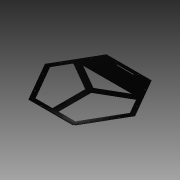
# Autodesk Inventor part: top
Saved by Autodesk Inventor 2015 SP1 (Build 190203100, 203)
## iProperties
Created: 2015-04-18
Part Number: top
Material: Ogólny
Document SubType Name: Konstrukcja blachowa
Designer: Marcin
Density: 1 g/cm^3
Sheet Metal Rule: Domyślny
Appearance: Gładki - czarny
Author: Marcin
Autodesk Inventor part; units mm, degrees
ref_plane "YZ Plane" through (0, 0, 0) normal (1, 0, 0) x (0, 1, 0)
ref_plane "XZ Plane" through (0, 0, 0) normal (0, 1, 0) x (-1, 0, 0)
ref_plane "XY Plane" through (0, 0, 0) normal (0, 0, 1) x (1, 0, 0)
sketch "Szkic1" plane through (0, 0, 0) normal (0, 0, 1) x (1, 0, 0)
  line L0 (76.2102, 132) -> (152.4205, 0)
  line L1 (152.4205, 0) -> (76.2102, -132)
  line L2 (76.2102, -132) -> (-76.2102, -132)
  line L3 (-76.2102, -132) -> (-152.4205, 0)
  line L4 (-152.4205, 0) -> (-76.2102, 132)
  line L5 (-76.2102, 132) -> (76.2102, 132)
  point P0 (0, 0)
  point P1 (0, 0)
  dimension "d0" = 132
  measures "d0" distance from line of L5 point (0, 0)
extrude "Płyta1" add sketch "Szkic1" along normal blind 0.8
sketch "Szkic2" plane through (0, 0, 0.8) normal (0, 0, 1) x (1, 0, 0)
  line L0 (152.4205, 0) -> (76.2102, -132) projected
  line L1 (76.2102, 132) -> (152.4205, 0) projected
  line L2 (-76.2102, 132) -> (76.2102, 132) projected
  line L3 (-152.4205, 0) -> (-76.2102, 132) projected
  line L4 (-76.2102, -132) -> (-152.4205, 0) projected
  line L5 (76.2102, -132) -> (-76.2102, -132) projected
  line L6 (0, 132) -> (0, -132) construction
  line L7 (-21.7321, -117) -> (-67.55, -117)
  line L8 (-67.55, -117) -> (-135.1, 0)
  line L9 (-36.5957, 60) -> (-100.4589, 60)
  line L10 (-100.4589, 60) -> (-135.1, 0)
  line L11 (-152.4205, 0) -> (-76.2102, 132) projected
  line L12 (21.7321, -117) -> (67.55, -117)
  line L13 (67.55, -117) -> (135.1, 0)
  line L14 (36.5957, 60) -> (100.4589, 60)
  line L15 (100.4589, 60) -> (135.1, 0)
  line L16 (-36.5957, 60) -> (0, 60)
  line L17 (0, 60) -> (36.5957, 60)
  line L18 (-21.7321, -117) -> (21.7321, -117)
  point P0 (0, 0)
  dimension "d5" = 15
  dimension "d6" = 15
  dimension "d7" = 15
  dimension "d14" = 177
  constraints: 24 end point, 5 symmetric about line, 4 parallel, 2 horizontal, 2 midpoint, 1 collinear, 1 point on line
  measures "d5" distance between parallel lines of L3 L10
  measures "d6" distance between parallel lines of L8 L4
  measures "d7" distance between parallel lines of L7 L5
  measures "d14" distance between parallel lines of L14 L12
extrude "Wytnij3" cut sketch "Szkic2" against normal blind 0.8 contours L7 L8 L10 L9 L16 L17 L14 L15 L13 L12 L18
sketch "Szkic3" plane through (0, 0, 0.8) normal (0, 0, 1) x (1, 0, 0)
  line L0 (135.1, 0) -> (67.55, -117)
  line L1 (-67.55, -117) -> (-135.1, 0)
  line L2 (67.55, -117) -> (-67.55, -117)
  line L3 (100.4589, 60) -> (135.1, 0)
  line L4 (-135.1, 0) -> (-100.4589, 60)
  line L5 (67.55, -117) -> (135.1, 0) construction
  line L6 (0, 0) -> (0, -117) construction
  line L7 (0, 0) -> (101.325, 58.5) construction
  line L8 (135.1, 0) -> (100.4589, 60) construction
  line L9 (0, 0) -> (-101.325, 58.5) construction
  line L10 (0, 0) -> (-101.325, 58.5) construction
  line L11 (5, 8.6603) -> (-96.325, 67.1603)
  line L12 (-106.325, 49.8397) -> (-5, -8.6603)
  arc A0 (-5, -8.6603) -> (5, 8.6603) centre (0, 0) ccw
  arc A1 (-96.325, 67.1603) -> (-106.325, 49.8397) centre (-101.325, 58.5) ccw
  line L13 (0, 0) -> (0, -117) construction
  line L14 (0, 0) -> (0, -117) construction
  line L15 (-10, 0) -> (-10, -117)
  line L16 (10, -117) -> (10, 0)
  arc A2 (10, 0) -> (-10, 0) centre (0, 0) ccw
  arc A3 (-10, -117) -> (10, -117) centre (0, -117) ccw
  line L17 (0, 0) -> (101.325, 58.5) construction
  line L18 (0, 0) -> (101.325, 58.5) construction
  line L19 (5, -8.6603) -> (106.325, 49.8397)
  line L20 (96.325, 67.1603) -> (-5, 8.6603)
  arc A4 (-5, 8.6603) -> (5, -8.6603) centre (0, 0) ccw
  arc A5 (106.325, 49.8397) -> (96.325, 67.1603) centre (101.325, 58.5) ccw
  point P0 (-50.6625, 29.25)
  point P1 (0, -58.5)
  point P2 (50.6625, 29.25)
  dimension "d15" = 20
  dimension "d18" = 240
  measures "d15" diameter of A1
sheet face with bend "Powierzchnia2" sketch "Szkic3" thickness 0.8 toward (0, 0, -1) bend radius 0.8 relief tear relief width 0.8 relief depth 0.4 contours L19 L16 A0 L11 L20 A5 | A3 L2 | L2 L15 L12 A0 L19 L16 | L19 A0 L16 | A0 A4 A2 | L20 A2 L15 L12 A1 L11 | L11 A2 L20 | L15 A4 L12
bend "Gięcie1"
sketch "Szkic5" plane through (0, 0, 0.8) normal (0, 0, 1) x (1, 0, 0)
  circle A0 centre (-128.0424, -30.624) radius 2 projected
  circle A1 centre (-90.5424, -95.576) radius 2 projected
  point P0 (0, 0)
  point P1 (-37.5, -126.2)
  point P2 (37.5, -126.2)
  point P3 (90.5424, -95.576)
  point P4 (128.0424, -30.624)
  point P5 (128.0424, 30.624)
  point P6 (90.5424, 95.576)
  point P7 (37.5, 126.2)
  point P8 (-37.5, 126.2)
  point P9 (-90.5424, 95.576)
  point P10 (-128.0424, 30.624)
  dimension "d38" = 360
  constraints: 2 coincident, 13 other
hole "Otwór3" at (-128.0424, -30.624, 0.8) at (-90.5424, -95.576, 0.8) at (-37.5, -126.2, 0.8) at (37.5, -126.2, 0.8) at (90.5424, -95.576, 0.8) at (128.0424, -30.624, 0.8) at (128.0424, 30.624, 0.8) at (90.5424, 95.576, 0.8) at (37.5, 126.2, 0.8) at (-37.5, 126.2, 0.8) at (-90.5424, 95.576, 0.8) at (-128.0424, 30.624, 0.8) direction (0, 0, -1) diameter 3 depth 0.8 tip angle 118
sketch "Szkic6" plane through (0, 0, 0.8) normal (0, 0, 1) x (1, 0, 0)
  line L0 (28.5, 120.2073) -> (-28.5, 120.2073) projected
  line L1 (-28.5, 120.2073) -> (-28.5, 118.2073) projected
  line L2 (28.5, 118.2073) -> (-28.5, 118.2073) projected
  line L3 (28.5, 120.2073) -> (28.5, 118.2073) projected
  line L4 (-29, 117.7073) -> (-29, 120.7073)
  line L5 (-29, 120.7073) -> (29, 120.7073)
  line L6 (29, 120.7073) -> (29, 117.7073)
  line L7 (29, 117.7073) -> (-29, 117.7073)
  point P0 (0, 0)
  dimension "d54" = 0.5
  constraints: 8 end point, 3 other
  measures "d54" distance between parallel lines of L1 L4
extrude "Wytnij4" cut sketch "Szkic6" against normal blind 0.8 contours L3 L2 L1 L0 | L4 L5 L6 L7
equation "\"d12\" = Grubość"
equation "\"d52\" = Grubość"
equation "\"d55\" = Grubość"
equation "\"d20\" = PromieńGięcia"
equation "\"d21\" = SzerokośćGięciaPodcięcia"
equation "\"d23\" = MinimalnaPozostałość"
equation "\"d22\" = GłębokośćGięciaPodcięcia"
equation "\"d24\" = PromieńGięcia"
equation "\"PromieńGięcia\" = Grubość"
equation "\"SzerokośćGięciaPodcięcia\" = Grubość"
equation "\"GłębokośćGięciaPodcięcia\" = 0.5 * Grubość"
equation "\"RozmiarPodcięciaNarożnika\" = 4 * Grubość"
equation "\"MinimalnaPozostałość\" = 2 * Grubość"
equation "\"PromieńPrzejścia\" = PromieńGięcia"
equation "\"Rozmiar_promienia_Jacobiego\" = Grubość"
equation "\"Wielk_odstępu\" = Grubość"
equation "\"d1\" = PromieńGięcia"
equation "\"Grubość\" = 0.8"
